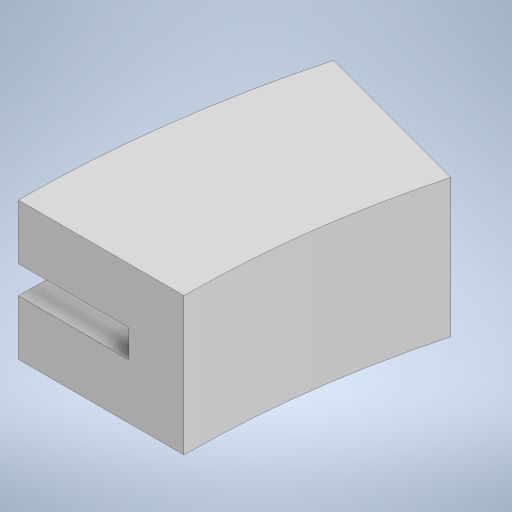
# Autodesk Inventor part: Moving Carousel Base Inner Clip
Saved by Autodesk Inventor 2023 (Build 270158000, 158)
## iProperties
Created: 2023-02-15
Part Number: Moving Carousel Base Inner Clip
Material: Generic
Document SubType Name: Modeling
Designer: cheng
Density: 1 g/cm^3
Appearance: Default
Author: cheng
Autodesk Inventor part; units mm, degrees
ref_plane "YZ Plane" through (0, 0, 0) normal (1, 0, 0) x (0, 1, 0)
ref_plane "XZ Plane" through (0, 0, 0) normal (0, 1, 0) x (-1, 0, 0)
ref_plane "XY Plane" through (0, 0, 0) normal (0, 0, 1) x (1, 0, 0)
sketch "Sketch1" plane through (0, 0, 0) normal (0, 1, 0) x (-1, 0, 0)
  circle A0 centre (0, 0) radius 165
  circle A1 centre (0, 0) radius 175
  line L0 (0, 0) -> (175, 0)
  line L1 (0, 0) -> (169.037, -45.2933)
  point P0 (159.3778, -42.7051)
  point P1 (165, 0)
  dimension "d0" = 10
  dimension "d1" = 330
  dimension "d2" = 15
  constraints: 4 end point, 2 centre point, 2 coincident, 2 point on circle, 1 horizontal
  measures "d0" radial gap between concentric circles of A0 A1
  measures "d1" diameter of A0
  measures "d2" angle of L1 L0
extrude "Extrusion1" add sketch "Sketch1" along normal blind 5 contours L0 A1 L1 A0 picked at (171.4447, -5.0841)
sketch "Sketch3" plane through (0, 5, 0) normal (0, 1, 0) x (1, 0, 0)
  arc A0 (-169.037, 45.2933) -> (-175, 0) centre (0, 0) ccw projected
  line L0 (-175, 0) -> (-165, 0) projected
  arc A1 (-159.3778, 42.7051) -> (-165, 0) centre (0, 0) ccw projected
  line L1 (-159.3778, 42.7051) -> (-169.037, 45.2933) projected
  circle A2 centre (0, 0) radius 175
  circle A3 centre (0, 0) radius 165
  circle A4 centre (0, 0) radius 195
  line L2 (0, 0) -> (-188.3555, 50.4697)
  line L3 (0, 0) -> (-195, 0)
  point P0 (-175, 0)
  dimension "d10" = 20
  constraints: 4 end point, 3 centre point, 3 coincident, 2 concentric, 2 point on circle, 1 horizontal
  measures "d10" radial gap between concentric circles of A0 A4
extrude "Extrusion2" add sketch "Sketch3" along normal blind 10 contours L1 A1 L0 A0 | A0 L3 A4 L2
sketch "Sketch4" plane through (0, 0, 0) normal (0, -1, 0) x (1, 0, 0)
  arc A0 (-195, 0) -> (-188.3555, -50.4697) centre (0, 0) ccw projected
  arc A1 (-175, 0) -> (-169.037, -45.2933) centre (0, 0) ccw projected
  line L0 (-159.3778, -42.7051) -> (-169.037, -45.2933) projected
  arc A2 (-165, 0) -> (-159.3778, -42.7051) centre (0, 0) ccw projected
  line L1 (-175, 0) -> (-165, 0) projected
  circle A3 centre (0, 0) radius 175
  circle A4 centre (0, 0) radius 195
  line L2 (0, 0) -> (-175, 0)
  line L3 (0, 0) -> (-169.037, -45.2933)
  arc A5 (-175, 0) -> (-169.037, -45.2933) centre (0, 0) ccw projected
  line L4 (-195, 0) -> (-175, 0) projected
  line L5 (-169.037, -45.2933) -> (-188.3555, -50.4697) projected
  point P0 (-169.037, -45.2933)
  constraints: 4 end point, 2 coincident, 1 centre point, 1 collinear, 1 concentric, 1 horizontal alignment, 3 other
extrude "Extrusion3" add sketch "Sketch4" along normal blind 10 contours L4 A1 L5 A0 | L1 A2 L0 A1
body "Solid1"
